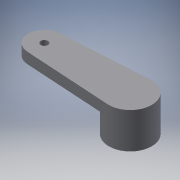
# Autodesk Inventor part: ServoArm
Saved by Autodesk Inventor 2018 (Build 220112000, 112)
## iProperties
Created: 2020-03-23
Part Number: ServoArm
Material: Generic
Document SubType Name: Modeling
Designer: technik
Density: 1 g/cm^3
Appearance: Default
Author: technik
Autodesk Inventor part; units mm, degrees
ref_plane "YZ Plane" through (0, 0, 0) normal (1, 0, 0) x (0, 1, 0)
ref_plane "XZ Plane" through (0, 0, 0) normal (0, 1, 0) x (-1, 0, 0)
ref_plane "XY Plane" through (0, 0, 0) normal (0, 0, 1) x (1, 0, 0)
sketch "Sketch1" plane through (0, 0, 0) normal (0, 0, 1) x (1, 0, 0)
  circle A0 centre (0, 0) radius 3
  dimension "d0" = 6
  constraints: 1 centre point, 1 coincident
  measures "d0" diameter of A0
extrude "Extrusion1" add sketch "Sketch1" along normal blind 5
sketch "Sketch2" plane through (0, 0, 5) normal (0, 0, 1) x (1, 0, 0)
  circle A0 centre (0, 0) radius 3 projected
  line L0 (0, 0) -> (-12, 0)
  circle A1 centre (-12, 0) radius 0.5
  circle A2 centre (-12, 0) radius 2.25
  line L1 (-0.1875, -2.9941) -> (-12.1406, -2.2456)
  line L2 (-12.1406, 2.2456) -> (-0.1875, 2.9941)
  circle A3 centre (0, 0) radius 3 projected
  dimension "d3" = 12
  dimension "d4" = 1
  dimension "d5" = 4.5
  constraints: 6 end point, 4 point on circle, 4 tangent, 2 centre point, 2 coincident, 1 horizontal
  measures "d3" distance of L0.start L0.end
  measures "d4" diameter of A1
  measures "d5" diameter of A2
extrude "Extrusion2" add sketch "Sketch2" against normal blind 1.5 contours A0 L0 A2 L2 | L1 A2 L0 A0 | A2
body "Solid1"
